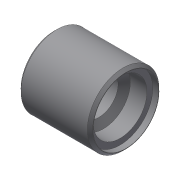
# Autodesk Inventor part: BELT_SUPPORT_OUTER
Saved by Autodesk Inventor 2019.4 (Build 234330000, 330)
## iProperties
Created: 2019-11-13
Part Number: BELT_SUPPORT_OUTER
Material: 一般
Document SubType Name: Modeling
Designer: y6tada
Density: 1 g/cm^3
Appearance: 既定
Author: y6tada
Autodesk Inventor part; units mm, degrees
ref_plane "YZ Plane" through (0, 0, 0) normal (1, 0, 0) x (0, 1, 0)
ref_plane "XZ Plane" through (0, 0, 0) normal (0, 1, 0) x (-1, 0, 0)
ref_plane "XY Plane" through (0, 0, 0) normal (0, 0, 1) x (1, 0, 0)
sketch "スケッチ1" plane through (0, 0, 0) normal (0, 0, 1) x (1, 0, 0)
  line L0 (-4, 4) -> (4, 4)
  line L1 (4, 4) -> (4, 2.15)
  line L2 (4, 2.15) -> (-4, 2.15)
  line L3 (-4, 2.15) -> (-4, 4)
  line L4 (0, 0) -> (0, 4.5155) construction
  line L5 (0, 0) -> (8.3877, 0) construction
  dimension "d0" = 8
  dimension "d1" = 4.3
  dimension "d2" = 8
  constraints: 12 end point, 2 horizontal, 2 parallel, 1 perpendicular, 1 vertical, 1 other
  measures "d0" distance of L0.start L0.end
  measures "d1" diameter of L2 L5
  measures "d2" diameter of L0 L5
revolve "回転1" add sketch "スケッチ1" angle 360 about axis through (0, 0, 0) along (1, 0, 0)
chamfer "面取り1" distance 0.3 angle 45 2 edges at (4, -4, 0) (-4, -4, 0)
sketch "スケッチ2" plane through (4, 0, 0) normal (1, 0, 0) x (0, 0, -1)
  point P0 (0, 0)
  point P1 (0, 0)
  constraints: 1 coincident
hole "穴1" at (4, 0, 0) direction (-1, 0, 0) diameter 6 depth 2.5 tip angle 118 counterbore diameter 7.3 counterbore depth 0.65
mirror "ミラー1" about plane through (0, 0, 0) normal (1, 0, 0) of "穴1"
